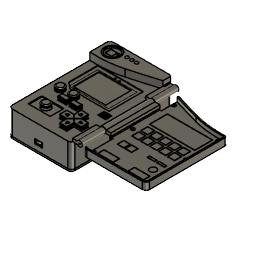
pokedexV4 (Autodesk Fusion 360 design; units mm, degrees)
part number: 2026-07-24-11-06-57-032
Autodesk Fusion 360 part; units mm, degrees
(part 1 of 3)
sketch "TubOutline" plane through (0, 0, 0) normal (0, 0, 1) x (1, 0, 0)
  line L0 (0, 0) -> (105, 0)
  line L1 (105, 0) -> (105, 170)
  line L2 (105, 170) -> (0, 170)
  line L3 (0, 170) -> (0, 0)
extrude "Extrude38" add sketch "TubOutline" against normal blind 44 makes body 1
fillet "Fillet13" radius 6 4 edges at (0, 0, -22) (105, 0, -22) (105, 170, -22) (0, 170, -22) on bodies 1
sketch "ShoulderStep" plane through (0, 0, 0) normal (0, 0, 1) x (1, 0, 0)
  arc A0 (0, 136) -> (54, 141) centre (11.7114, 303.6168) ccw
  arc A1 (54, 141) -> (105, 156) centre (-358, 1636) ccw
  line L0 (105, 156) -> (105, 0)
  line L1 (105, 0) -> (0, 0)
  line L2 (0, 0) -> (0, 136)
extrude "Extrude39" cut sketch "ShoulderStep" against normal blind 4 bodies 1
shell "Shell6" thickness 2.4 removed faces 1 at (35, 111.3333, -44) on bodies 1
ref_plane "WorkPlane4" through (0, 0, -4) normal (0, 0, 1) x (1, 0, 0)
sketch "FaceCuts" plane through (0, 0, -4) normal (0, 0, 1) x (1, 0, 0)
  line L0 (21.2, 84.4) -> (78.8, 84.4)
  line L1 (78.8, 84.4) -> (78.8, 127.6)
  line L2 (78.8, 127.6) -> (21.2, 127.6)
  line L3 (21.2, 127.6) -> (21.2, 84.4)
  line L4 (12.7, 75.9) -> (87.3, 75.9)
  line L5 (87.3, 75.9) -> (87.3, 136.1)
  line L6 (87.3, 136.1) -> (12.7, 136.1)
  line L7 (12.7, 136.1) -> (12.7, 75.9)
  circle A0 centre (17.5, 69) radius 7.2
  line L8 (65.5, 63) -> (88.5, 63)
  line L9 (88.5, 63) -> (88.5, 64.5)
  line L10 (88.5, 64.5) -> (65.5, 64.5)
  line L11 (65.5, 64.5) -> (65.5, 63)
  line L12 (65.5, 66) -> (88.5, 66)
  line L13 (88.5, 66) -> (88.5, 67.5)
  line L14 (88.5, 67.5) -> (65.5, 67.5)
  line L15 (65.5, 67.5) -> (65.5, 66)
  line L16 (65.5, 69) -> (88.5, 69)
  line L17 (88.5, 69) -> (88.5, 70.5)
  line L18 (88.5, 70.5) -> (65.5, 70.5)
  line L19 (65.5, 70.5) -> (65.5, 69)
  line L20 (65.5, 72) -> (88.5, 72)
  line L21 (88.5, 72) -> (88.5, 73.5)
  line L22 (88.5, 73.5) -> (65.5, 73.5)
  line L23 (65.5, 73.5) -> (65.5, 72)
  line L24 (65.5, 75) -> (88.5, 75)
  line L25 (88.5, 75) -> (88.5, 76.5)
  line L26 (88.5, 76.5) -> (65.5, 76.5)
  line L27 (65.5, 76.5) -> (65.5, 75)
  line L28 (65.5, 78) -> (88.5, 78)
  line L29 (88.5, 78) -> (88.5, 79.5)
  line L30 (88.5, 79.5) -> (65.5, 79.5)
  line L31 (65.5, 79.5) -> (65.5, 78)
  line L32 (65.5, 81) -> (88.5, 81)
  line L33 (88.5, 81) -> (88.5, 82.5)
  line L34 (88.5, 82.5) -> (65.5, 82.5)
  line L35 (65.5, 82.5) -> (65.5, 81)
  line L36 (30.5, 54) -> (45.5, 54)
  line L37 (45.5, 54) -> (45.5, 58)
  line L38 (45.5, 58) -> (30.5, 58)
  line L39 (30.5, 58) -> (30.5, 54)
  line L40 (49.5, 54) -> (64.5, 54)
  line L41 (64.5, 54) -> (64.5, 58)
  line L42 (64.5, 58) -> (49.5, 58)
  line L43 (49.5, 58) -> (49.5, 54)
  line L44 (11.5, 21) -> (48.5, 21)
  line L45 (48.5, 21) -> (48.5, 44)
  line L46 (48.5, 44) -> (11.5, 44)
  line L47 (11.5, 44) -> (11.5, 21)
  line L48 (71.3, 13.5) -> (83.7, 13.5)
  line L49 (83.7, 13.5) -> (83.7, 50.5)
  line L50 (83.7, 50.5) -> (71.3, 50.5)
  line L51 (71.3, 50.5) -> (71.3, 13.5)
  line L52 (59, 25.8) -> (96, 25.8)
  line L53 (96, 25.8) -> (96, 38.2)
  line L54 (96, 38.2) -> (59, 38.2)
  line L55 (59, 38.2) -> (59, 25.8)
extrude "Extrude40" cut sketch "FaceCuts" against normal blind 1.6 contours L0 L1 L2 L3 | L4 L5 L6 L7 A0 L26 L27 L28 L30 L31 L32 L34 L35 bodies 1
extrude "Extrude41" cut sketch "FaceCuts" against normal blind 6 contours L0 L1 L2 L3 bodies 1
extrude "Extrude42" cut sketch "FaceCuts" against normal blind 6 contours L4 A0 picked at (17.378, 71.2031) bodies 1
extrude "Extrude43" cut sketch "FaceCuts" against normal blind 6 contours L4 L5 L26 L27 | L4 L5 L24 L25 L26 L27 | L5 L32 L33 L34 | L5 L32 L34 L35 | L5 L28 L29 L30 | L5 L28 L30 L31 | L8 L9 L10 L11 | L12 L13 L14 L15 | L16 L17 L18 L19 | L20 L21 L22 L23 bodies 1
extrude "Extrude44" cut sketch "FaceCuts" against normal blind 6 contours L36 L37 L38 L39 | L40 L41 L42 L43 bodies 1
extrude "Extrude45" cut sketch "FaceCuts" against normal blind 1.6 contours L44 L45 L46 L47 bodies 1
extrude "Extrude46" cut sketch "FaceCuts" against normal blind 6 contours L48 L49 L51 L52 | L51 L52 L54 L55 | L49 L51 L52 L54 | L49 L52 L53 L54 | L49 L50 L51 L54 bodies 1
sketch "ShoulderDetail" plane through (0, 0, 0) normal (0, 0, 1) x (1, 0, 0)
  circle A0 centre (19, 155) radius 13.5
  circle A1 centre (39, 159.5) radius 2.8
  circle A2 centre (47, 159.5) radius 2.8
  circle A3 centre (55, 159.5) radius 2.8
extrude "Extrude47" cut sketch "ShoulderDetail" against normal blind 2.2 contours A0 bodies 1
extrude "Extrude48" cut sketch "ShoulderDetail" against normal blind 8 contours A1 | A2 | A3 bodies 1
ref_plane "WorkPlane5" through (0, 0, -6.4) normal (0, 0, 1) x (1, 0, 0)
sketch "PlateBosses" plane through (0, 0, -6.4) normal (0, 0, 1) x (1, 0, 0)
  circle A0 centre (11.5, 11.5) radius 4.2
  circle A1 centre (11.5, 85) radius 4.2
  circle A2 centre (11.5, 156) radius 4.2
  circle A3 centre (93, 11.5) radius 4.2
  circle A4 centre (93, 80) radius 4.2
  circle A5 centre (93, 120) radius 4.2
extrude "Extrude51" add sketch "PlateBosses" against normal blind 37.6 bodies 1 makes body 2 at (14.7174, 158.6997, -31.4667)
sketch "PlatePilots" plane through (0, 0, -6.4) normal (0, 0, 1) x (1, 0, 0)
  circle A0 centre (11.5, 11.5) radius 1.25
  circle A1 centre (11.5, 85) radius 1.25
  circle A2 centre (11.5, 156) radius 1.25
  circle A3 centre (93, 11.5) radius 1.25
  circle A4 centre (93, 80) radius 1.25
  circle A5 centre (93, 120) radius 1.25
extrude "Extrude52" cut sketch "PlatePilots" against normal blind 12 from surface at -26 bodies 1
sketch "USBC" plane through (0, 0, 0) normal (0, 1, 0) x (1, 0, 0)
  line L0 (45.5, 28) -> (54.5, 28)
  line L1 (54.5, 28) -> (54.5, 31.5)
  line L2 (54.5, 31.5) -> (45.5, 31.5)
  line L3 (45.5, 31.5) -> (45.5, 28)
extrude "Extrude53" cut sketch "USBC" along normal mid plane 16 bodies 1
ref_plane "WorkPlane6" through (0, 0, -44) normal (0, 0, 1) x (1, 0, 0)
sketch "PlateOutline" plane through (0, 0, -44) normal (0, 0, 1) x (1, 0, 0)
  line L0 (0, 0) -> (105, 0)
  line L1 (105, 0) -> (105, 170)
  line L2 (105, 170) -> (0, 170)
  line L3 (0, 170) -> (0, 0)
extrude "Extrude60" add sketch "PlateOutline" against normal blind 3 separate body makes body 3
fillet "Fillet15" radius 6 4 edges at (0, 0, -45.5) (105, 0, -45.5) (105, 170, -45.5) (0, 170, -45.5) on bodies 3
sketch "PlateFeatures" plane through (0, 0, -44) normal (0, 0, 1) x (1, 0, 0)
  circle A0 centre (11.5, 11.5) radius 1.6
  circle A1 centre (11.5, 85) radius 1.6
  circle A2 centre (11.5, 156) radius 1.6
  circle A3 centre (93, 11.5) radius 1.6
  circle A4 centre (93, 80) radius 1.6
  circle A5 centre (93, 120) radius 1.6
  circle A6 centre (52, 132) radius 21
  line L0 (47.5, 127.5) -> (56.5, 127.5)
  line L1 (56.5, 127.5) -> (56.5, 136.5)
  line L2 (56.5, 136.5) -> (47.5, 136.5)
  line L3 (47.5, 136.5) -> (47.5, 127.5)
extrude "Extrude61" cut sketch "PlateFeatures" against normal blind 4 contours A0 | A1 | A2 | A3 | A4 | A5 bodies 3
extrude "Extrude62" cut sketch "PlateFeatures" against normal blind 1 contours A6 bodies 3
extrude "Extrude63" cut sketch "PlateFeatures" against normal blind 4 contours L0 L1 L2 L3 bodies 3
sketch "BossBridge" plane through (0, 0, 0) normal (0, 0, 1) x (1, 0, 0)
  circle A0 centre (11.5, 156) radius 4.2
extrude "Extrude66" add sketch "BossBridge" against normal blind 5 from surface at -2 bodies 1 2
sketch "FillVoids" plane through (0, 0, 0) normal (0, 0, 1) x (1, 0, 0)
  circle A0 centre (19, 155) radius 13.5
  circle A1 centre (39, 159.5) radius 2.8
  circle A2 centre (47, 159.5) radius 2.8
  circle A3 centre (55, 159.5) radius 2.8
extrude "Extrude75" add sketch "FillVoids" along normal blind 8 from surface at -8 bodies 1
sketch "ShoulderRaise" plane through (0, 0, 0) normal (0, 0, 1) x (1, 0, 0)
  arc A0 (0, 136) -> (54, 141) centre (11.7114, 303.6168) ccw
  arc A1 (54, 141) -> (105, 156) centre (-358, 1636) ccw
  line L0 (105, 156) -> (105, 164)
  arc A2 (105, 164) -> (99, 170) centre (98.991, 163.991) ccw
  line L1 (99, 170) -> (6, 170)
  arc A3 (6, 170) -> (0, 164) centre (6.009, 163.991) ccw
  line L2 (0, 164) -> (0, 136)
extrude "Extrude76" add sketch "ShoulderRaise" along normal blind 8 bodies 1
ref_plane "WorkPlane7" through (0, 0, 8) normal (0, 0, 1) x (1, 0, 0)
sketch "ShoulderDetail2" plane through (0, 0, 8) normal (0, 0, 1) x (1, 0, 0)
  circle A0 centre (19, 155) radius 13.5
  circle A1 centre (39, 159.5) radius 2.8
  circle A2 centre (47, 159.5) radius 2.8
  circle A3 centre (55, 159.5) radius 2.8
extrude "Extrude77" cut sketch "ShoulderDetail2" against normal blind 2.2 contours A0 bodies 1
extrude "Extrude78" cut sketch "ShoulderDetail2" against normal blind 16 contours A1 | A2 | A3 bodies 1
sketch "SwingRelief" plane through (0, 0, 0) normal (0, 1, 0) x (1, 0, 0)
  line L0 (103.2, -8.5) -> (105.5, -8.5)
  line L1 (105.5, -8.5) -> (105.5, -0.5)
  line L2 (105.5, -0.5) -> (103.2, -0.5)
  line L3 (103.2, -0.5) -> (103.2, -8.5)
extrude "Extrude88" cut sketch "SwingRelief" along normal blind 42 from surface at 128 bodies 1
sketch "LidOutline" plane through (0, 0, 0) normal (0, 0, 1) x (1, 0, 0)
  arc A0 (125, 156) -> (176, 141) centre (588, 1636) ccw
  arc A1 (176, 141) -> (230, 136) centre (218.2886, 303.6168) ccw
  line L0 (230, 136) -> (230, 0)
  line L1 (230, 0) -> (125, 0)
  line L2 (125, 0) -> (125, 156)
extrude "Extrude89" add sketch "LidOutline" against normal blind 12 separate body makes body 4
fillet "Fillet19" radius 6 2 edges at (230, 0, -6) (125, 0, -6) on bodies 4
fillet "Fillet20" radius 3 1 edges at (230, 136, -6) on bodies 4
shell "Shell10" thickness 2.4 removed faces 1 at (182.5811, 49.8482, 0) on bodies 4
ref_plane "WorkPlane8" through (0, 0, -2) normal (0, 0, 1) x (1, 0, 0)
sketch "LidBosses" plane through (0, 0, -2) normal (0, 0, 1) x (1, 0, 0)
  circle A0 centre (133, 9) radius 3.2
  circle A1 centre (133, 75) radius 3.2
  circle A2 centre (133, 144) radius 3.2
  circle A3 centre (222, 9) radius 3.2
  circle A4 centre (222, 75) radius 3.2
  circle A5 centre (222, 129) radius 3.2
extrude "Extrude95" add sketch "LidBosses" against normal blind 10 bodies 4
sketch "LidInsertBores" plane through (0, 0, -2) normal (0, 0, 1) x (1, 0, 0)
  circle A0 centre (133, 9) radius 1.6
  circle A1 centre (133, 75) radius 1.6
  circle A2 centre (133, 144) radius 1.6
  circle A3 centre (222, 9) radius 1.6
  circle A4 centre (222, 75) radius 1.6
  circle A5 centre (222, 129) radius 1.6
extrude "Extrude96" cut sketch "LidInsertBores" against normal blind 4.5 bodies 4
sketch "FacePlateOutline" plane through (0, 0, 0) normal (0, 0, 1) x (1, 0, 0)
  arc A0 (127.9, 152.5) -> (176, 138.5) centre (719.1151, 2094.1174) ccw
  arc A1 (176, 138.5) -> (227.1, 133.5) centre (217.0513, 294.4236) ccw
  line L0 (227.1, 133.5) -> (227.1, 2.9)
  line L1 (227.1, 2.9) -> (127.9, 2.9)
  line L2 (127.9, 2.9) -> (127.9, 152.5)
extrude "Extrude97" add sketch "FacePlateOutline" along normal blind 2 from surface at -2 separate body makes body 5
sketch "FacePlateCuts" plane through (0, 0, 0) normal (0, 0, 1) x (1, 0, 0)
  line L0 (140, 96) -> (216, 96)
  line L1 (216, 96) -> (216, 126)
  line L2 (216, 126) -> (140, 126)
  line L3 (140, 126) -> (140, 96)
  line L4 (142, 79) -> (154, 79)
  line L5 (154, 79) -> (154, 91)
  line L6 (154, 91) -> (142, 91)
  line L7 (142, 91) -> (142, 79)
  line L8 (157, 79) -> (169, 79)
  line L9 (169, 79) -> (169, 91)
  line L10 (169, 91) -> (157, 91)
  line L11 (157, 91) -> (157, 79)
  line L12 (172, 79) -> (184, 79)
  line L13 (184, 79) -> (184, 91)
  line L14 (184, 91) -> (172, 91)
  line L15 (172, 91) -> (172, 79)
  line L16 (187, 79) -> (199, 79)
  line L17 (199, 79) -> (199, 91)
  line L18 (199, 91) -> (187, 91)
  line L19 (187, 91) -> (187, 79)
  line L20 (202, 79) -> (214, 79)
  line L21 (214, 79) -> (214, 91)
  line L22 (214, 91) -> (202, 91)
  line L23 (202, 91) -> (202, 79)
  line L24 (142, 64) -> (154, 64)
  line L25 (154, 64) -> (154, 76)
  line L26 (154, 76) -> (142, 76)
  line L27 (142, 76) -> (142, 64)
  line L28 (157, 64) -> (169, 64)
  line L29 (169, 64) -> (169, 76)
  line L30 (169, 76) -> (157, 76)
  line L31 (157, 76) -> (157, 64)
  line L32 (172, 64) -> (184, 64)
  line L33 (184, 64) -> (184, 76)
  line L34 (184, 76) -> (172, 76)
  line L35 (172, 76) -> (172, 64)
  line L36 (187, 64) -> (199, 64)
  line L37 (199, 64) -> (199, 76)
  line L38 (199, 76) -> (187, 76)
  line L39 (187, 76) -> (187, 64)
  line L40 (202, 64) -> (214, 64)
  line L41 (214, 64) -> (214, 76)
  line L42 (214, 76) -> (202, 76)
  line L43 (202, 76) -> (202, 64)
  line L44 (142, 40) -> (153, 40)
  line L45 (153, 40) -> (153, 51)
  line L46 (153, 51) -> (142, 51)
  line L47 (142, 51) -> (142, 40)
  line L48 (155, 40) -> (166, 40)
  line L49 (166, 40) -> (166, 51)
  line L50 (166, 51) -> (155, 51)
  line L51 (155, 51) -> (155, 40)
  line L52 (186, 46) -> (199, 46)
  line L53 (199, 46) -> (199, 50)
  line L54 (199, 50) -> (186, 50)
  line L55 (186, 50) -> (186, 46)
  line L56 (202, 46) -> (215, 46)
  line L57 (215, 46) -> (215, 50)
  line L58 (215, 50) -> (202, 50)
  line L59 (202, 50) -> (202, 46)
  circle A0 centre (209, 33) radius 5.5
  line L60 (139, 10) -> (165, 10)
  line L61 (165, 10) -> (165, 21)
  line L62 (165, 21) -> (139, 21)
  line L63 (139, 21) -> (139, 10)
  line L64 (190, 10) -> (216, 10)
  line L65 (216, 10) -> (216, 21)
  line L66 (216, 21) -> (190, 21)
  line L67 (190, 21) -> (190, 10)
  circle A1 centre (133, 9) radius 1.15
  circle A2 centre (133, 75) radius 1.15
  circle A3 centre (133, 144) radius 1.15
  circle A4 centre (222, 9) radius 1.15
  circle A5 centre (222, 75) radius 1.15
  circle A6 centre (222, 129) radius 1.15
extrude "Extrude98" cut sketch "FacePlateCuts" along normal blind 3 from surface at -2.5 bodies 5
ref_plane "WorkPlane9" through (0, 0, -44) normal (0, 0, 1) x (1, 0, 0)
sketch "M3Bores" plane through (0, 0, -44) normal (0, 0, 1) x (1, 0, 0)
  circle A0 centre (11.5, 11.5) radius 2
  circle A1 centre (11.5, 85) radius 2
  circle A2 centre (11.5, 156) radius 2
  circle A3 centre (93, 11.5) radius 2
  circle A4 centre (93, 80) radius 2
  circle A5 centre (93, 120) radius 2
extrude "Extrude99" cut sketch "M3Bores" along normal blind 6.5 bodies 1
sketch "M3Clear" plane through (0, 0, -44) normal (0, 0, 1) x (1, 0, 0)
  circle A0 centre (11.5, 11.5) radius 1.7
  circle A1 centre (11.5, 85) radius 1.7
  circle A2 centre (11.5, 156) radius 1.7
  circle A3 centre (93, 11.5) radius 1.7
  circle A4 centre (93, 80) radius 1.7
  circle A5 centre (93, 120) radius 1.7
extrude "Extrude100" cut sketch "M3Clear" against normal blind 4 bodies 3
sketch "LidNotches" plane through (0, 0, 0) normal (0, 0, 1) x (1, 0, 0)
  line L0 (124.5, 3) -> (130.5, 3)
  line L1 (130.5, 3) -> (130.5, 44.5)
  line L2 (130.5, 44.5) -> (124.5, 44.5)
  line L3 (124.5, 44.5) -> (124.5, 3)
  line L4 (124.5, 125.5) -> (130.5, 125.5)
  line L5 (130.5, 125.5) -> (130.5, 157)
  line L6 (130.5, 157) -> (124.5, 157)
  line L7 (124.5, 157) -> (124.5, 125.5)
extrude "Extrude108" cut sketch "LidNotches" against normal blind 16 from surface at 2 bodies 4
extrude "Extrude109" cut sketch "LidNotches" against normal blind 3 from surface at 0.5 bodies 5
sketch "SpineTrim" plane through (0, 0, 0) normal (0, 1, 0) x (1, 0, 0)
  line L0 (103.5, 0) -> (105.5, 0)
  line L1 (105.5, 0) -> (105.5, 2.5)
  line L2 (105.5, 2.5) -> (103.5, 2.5)
  line L3 (103.5, 2.5) -> (103.5, 0)
extrude "Extrude110" cut sketch "SpineTrim" along normal blind 156 from surface at 4 bodies 1
sketch "WindowEnlarge" plane through (0, 0, 0) normal (0, 0, 1) x (1, 0, 0)
  line L0 (20.7, 83.9) -> (79.3, 83.9)
  line L1 (79.3, 83.9) -> (79.3, 128.1)
  line L2 (79.3, 128.1) -> (20.7, 128.1)
  line L3 (20.7, 128.1) -> (20.7, 83.9)
extrude "Extrude111" cut sketch "WindowEnlarge" against normal blind 8 bodies 1
sketch "LCDPocketRibs" plane through (0, 0, -6.4) normal (0, 0, 1) x (1, 0, 0)
  line L0 (15.95, 78.55) -> (18.95, 78.55)
  line L1 (18.95, 78.55) -> (18.95, 130.45)
  line L2 (18.95, 130.45) -> (15.95, 130.45)
  line L3 (15.95, 130.45) -> (15.95, 78.55)
  line L4 (85.65, 78.55) -> (88.65, 78.55)
  line L5 (88.65, 78.55) -> (88.65, 130.45)
  line L6 (88.65, 130.45) -> (85.65, 130.45)
  line L7 (85.65, 130.45) -> (85.65, 78.55)
  line L8 (15.95, 78.55) -> (88.65, 78.55)
  line L9 (88.65, 78.55) -> (88.65, 81.55)
  line L10 (88.65, 81.55) -> (15.95, 81.55)
  line L11 (15.95, 81.55) -> (15.95, 78.55)
  line L12 (15.95, 139.05) -> (27.95, 139.05)
  line L13 (27.95, 139.05) -> (27.95, 142.05)
  line L14 (27.95, 142.05) -> (15.95, 142.05)
  line L15 (15.95, 142.05) -> (15.95, 139.05)
  line L16 (76.65, 139.05) -> (88.65, 139.05)
  line L17 (88.65, 139.05) -> (88.65, 142.05)
  line L18 (88.65, 142.05) -> (76.65, 142.05)
  line L19 (76.65, 142.05) -> (76.65, 139.05)
extrude "Extrude112" add sketch "LCDPocketRibs" against normal blind 10 bodies 1
sketch "ClampPedestals" plane through (0, 0, -6.4) normal (0, 0, 1) x (1, 0, 0)
  circle A0 centre (11.5, 106) radius 4
  circle A1 centre (93.5, 106) radius 4
extrude "Extrude113" add sketch "ClampPedestals" against normal blind 8 bodies 1
sketch "ClampInsertBores" plane through (0, 0, -6.4) normal (0, 0, 1) x (1, 0, 0)
  circle A0 centre (11.5, 106) radius 1.6
  circle A1 centre (93.5, 106) radius 1.6
extrude "Extrude114" cut sketch "ClampInsertBores" against normal blind 4.5 from surface at -3.5 bodies 1
ref_plane "WorkPlane10" through (0, 0, -14.4) normal (0, 0, 1) x (1, 0, 0)
ref_plane "WorkPlane11" through (0, 0, -13.6) normal (0, 0, 1) x (1, 0, 0)
sketch "CrossPlateOutline" plane through (0, 0, -13.6) normal (0, 0, 1) x (1, 0, 0)
  line L0 (16, 105.5) -> (88.6, 105.5)
  line L1 (88.6, 105.5) -> (88.6, 139.5)
  line L2 (88.6, 139.5) -> (16, 139.5)
  line L3 (16, 139.5) -> (16, 105.5)
extrude "Extrude117" add sketch "CrossPlateOutline" against normal blind 2.5 separate body makes body 6
sketch "CrossPlateCuts" plane through (0, 0, -13.6) normal (0, 0, 1) x (1, 0, 0)
  circle A0 centre (24.05, 134.1) radius 2.8
  circle A1 centre (82.05, 134.1) radius 2.8
  circle A2 centre (24.05, 111.1) radius 2.8
  circle A3 centre (82.05, 111.1) radius 2.8
  line L0 (33, 107.5) -> (73, 107.5)
  line L1 (73, 107.5) -> (73, 137.5)
  line L2 (73, 137.5) -> (33, 137.5)
  line L3 (33, 137.5) -> (33, 107.5)
extrude "Extrude118" cut sketch "CrossPlateCuts" against normal blind 3 bodies 6
sketch "PedestalExtend" plane through (0, 0, -6.4) normal (0, 0, 1) x (1, 0, 0)
  circle A0 centre (11.5, 106) radius 4
  circle A1 centre (93.5, 106) radius 4
extrude "Extrude119" add sketch "PedestalExtend" against normal blind 10 bodies 1
sketch "PedestalBores2" plane through (0, 0, -6.4) normal (0, 0, 1) x (1, 0, 0)
  circle A0 centre (11.5, 106) radius 1.6
  circle A1 centre (93.5, 106) radius 1.6
extrude "Extrude120" cut sketch "PedestalBores2" against normal blind 4.5 from surface at -5.5 bodies 1
sketch "PlateEars" plane through (0, 0, -13.6) normal (0, 0, 1) x (1, 0, 0)
  line L0 (7, 101) -> (16.2, 101)
  line L1 (16.2, 101) -> (16.2, 111)
  line L2 (16.2, 111) -> (7, 111)
  line L3 (7, 111) -> (7, 101)
  line L4 (88.4, 101) -> (98, 101)
  line L5 (98, 101) -> (98, 111)
  line L6 (98, 111) -> (88.4, 111)
  line L7 (88.4, 111) -> (88.4, 101)
extrude "Extrude121" add sketch "PlateEars" against normal blind 2.5 bodies 6
sketch "EarHoles" plane through (0, 0, -13.6) normal (0, 0, 1) x (1, 0, 0)
  circle A0 centre (11.5, 106) radius 1.15
  circle A1 centre (93.5, 106) radius 1.15
extrude "Extrude122" cut sketch "EarHoles" against normal blind 3 bodies 6
sketch "HoleFill" plane through (0, 0, -13.6) normal (0, 0, 1) x (1, 0, 0)
  circle A0 centre (24.05, 134.1) radius 2.85
  circle A1 centre (82.05, 134.1) radius 2.85
  circle A2 centre (24.05, 111.1) radius 2.85
  circle A3 centre (82.05, 111.1) radius 2.85
extrude "Extrude123" add sketch "HoleFill" against normal blind 2.5 bodies 6
sketch "M25Holes" plane through (0, 0, -13.6) normal (0, 0, 1) x (1, 0, 0)
  circle A0 centre (24.05, 134.1) radius 1.35
  circle A1 centre (82.05, 134.1) radius 1.35
  circle A2 centre (24.05, 111.1) radius 1.35
  circle A3 centre (82.05, 111.1) radius 1.35
extrude "Extrude124" cut sketch "M25Holes" against normal blind 3 bodies 6
sketch "HingeTub" plane through (0, 0, 0) normal (0, 1, 0) x (1, 0, 0)
  circle A0 centre (115, 2) radius 4.5
  line L0 (103, 0) -> (115, 0)
  line L1 (115, 0) -> (115, 5)
  line L2 (115, 5) -> (103, 5)
  line L3 (103, 5) -> (103, 0)
extrude "Extrude125" add sketch "HingeTub" along normal blind 39.7 from surface at 4 bodies 1
extrude "Extrude126" add sketch "HingeTub" along normal blind 39.7 from surface at 126.3 bodies 1
sketch "HingeLid" plane through (0, 0, 0) normal (0, 1, 0) x (1, 0, 0)
  circle A0 centre (115, 2) radius 4.5
  line L0 (115, 0) -> (128, 0)
  line L1 (128, 0) -> (128, 5)
  line L2 (128, 5) -> (115, 5)
  line L3 (115, 5) -> (115, 0)
extrude "Extrude127" add sketch "HingeLid" along normal blind 82 from surface at 44 bodies 4
sketch "PinBore" plane through (0, 0, 0) normal (0, 1, 0) x (1, 0, 0)
  circle A0 centre (115, 2) radius 1
extrude "Extrude128" cut sketch "PinBore" along normal blind 162 from surface at 4 bodies 1 4
sketch "FlushCleanup" plane through (0, 0, -13.6) normal (0, 0, 1) x (1, 0, 0)
  line L0 (15, 78) -> (89, 78)
  line L1 (89, 78) -> (89, 140)
  line L2 (89, 140) -> (15, 140)
  line L3 (15, 140) -> (15, 78)
extrude "Extrude129" cut sketch "FlushCleanup" against normal blind 8 bodies 1
sketch "PedestalBoresFlush" plane through (0, 0, -13.6) normal (0, 0, 1) x (1, 0, 0)
  circle A0 centre (11.5, 106) radius 1.6
  circle A1 centre (93.5, 106) radius 1.6
extrude "Extrude130" cut sketch "PedestalBoresFlush" along normal blind 4.5 bodies 1
ref_plane "WorkPlane12" through (0, 0, -5.6) normal (0, 0, 1) x (1, 0, 0)
sketch "DisplayDummySk" plane through (0, 0, -5.6) normal (0, 0, 1) x (1, 0, 0)
  line L0 (19.45, 82.05) -> (85.15, 82.05)
  line L1 (85.15, 82.05) -> (85.15, 129.95)
  line L2 (85.15, 129.95) -> (19.45, 129.95)
  line L3 (19.45, 129.95) -> (19.45, 82.05)
extrude "Extrude132" add sketch "DisplayDummySk" against normal blind 8 separate body makes body 7
sketch "KnuckleGap" plane through (0, 0, 0) normal (0, 1, 0) x (1, 0, 0)
  line L0 (109, -8) -> (124.9, -8)
  line L1 (124.9, -8) -> (124.9, 8)
  line L2 (124.9, 8) -> (109, 8)
  line L3 (109, 8) -> (109, -8)
extrude "Extrude133" cut sketch "KnuckleGap" along normal blind 16 from surface at 77 bodies 4
sketch "WireSlot" plane through (0, 0, 0) normal (1, 0, 0) x (0, 0, -1)
  line L0 (3, 79.5) -> (11, 79.5)
  line L1 (11, 79.5) -> (11, 90.5)
  line L2 (11, 90.5) -> (3, 90.5)
  line L3 (3, 90.5) -> (3, 79.5)
extrude "Extrude134" cut sketch "WireSlot" along normal blind 6 from surface at 102 bodies 1
extrude "Extrude135" cut sketch "WireSlot" along normal blind 6 from surface at 124 bodies 4
sketch "PokeballFill" plane through (0, 0, -44) normal (0, 0, 1) x (1, 0, 0)
  circle A0 centre (52, 132) radius 21
  line L0 (47.5, 127.5) -> (56.5, 127.5)
  line L1 (56.5, 127.5) -> (56.5, 136.5)
  line L2 (56.5, 136.5) -> (47.5, 136.5)
  line L3 (47.5, 136.5) -> (47.5, 127.5)
extrude "Extrude138" add sketch "PokeballFill" against normal blind 1 bodies 3
ref_plane "WorkPlane13" through (0, 0, -47) normal (0, 0, 1) x (1, 0, 0)
sketch "PokeballOuter" plane through (0, 0, -47) normal (0, 0, 1) x (1, 0, 0)
  circle A0 centre (52, 132) radius 21
  line L0 (47.5, 127.5) -> (56.5, 127.5)
  line L1 (56.5, 127.5) -> (56.5, 136.5)
  line L2 (56.5, 136.5) -> (47.5, 136.5)
  line L3 (47.5, 136.5) -> (47.5, 127.5)
extrude "Extrude139" cut sketch "PokeballOuter" along normal blind 1 bodies 3
sketch "RingRibs" plane through (0, 0, -47) normal (0, 0, 1) x (1, 0, 0)
  circle A0 centre (52, 132) radius 21
  line L0 (47.5, 127.5) -> (56.5, 127.5)
  line L1 (56.5, 127.5) -> (56.5, 136.5)
  line L2 (56.5, 136.5) -> (47.5, 136.5)
  line L3 (47.5, 136.5) -> (47.5, 127.5)
  line L4 (29, 137.6) -> (75, 137.6)
  line L5 (75, 137.6) -> (75, 139.2)
  line L6 (75, 139.2) -> (29, 139.2)
  line L7 (29, 139.2) -> (29, 137.6)
  line L8 (29, 140.8) -> (75, 140.8)
  line L9 (75, 140.8) -> (75, 142.4)
  line L10 (75, 142.4) -> (29, 142.4)
  line L11 (29, 142.4) -> (29, 140.8)
  line L12 (29, 144) -> (75, 144)
  line L13 (75, 144) -> (75, 145.6)
  line L14 (75, 145.6) -> (29, 145.6)
  line L15 (29, 145.6) -> (29, 144)
  line L16 (29, 147.2) -> (75, 147.2)
  line L17 (75, 147.2) -> (75, 148.8)
  line L18 (75, 148.8) -> (29, 148.8)
  line L19 (29, 148.8) -> (29, 147.2)
  line L20 (29, 150.4) -> (75, 150.4)
  line L21 (75, 150.4) -> (75, 152)
  line L22 (75, 152) -> (29, 152)
  line L23 (29, 152) -> (29, 150.4)
  line L24 (29, 124.8) -> (75, 124.8)
  line L25 (75, 124.8) -> (75, 126.4)
  line L26 (75, 126.4) -> (29, 126.4)
  line L27 (29, 126.4) -> (29, 124.8)
  line L28 (29, 121.6) -> (75, 121.6)
  line L29 (75, 121.6) -> (75, 123.2)
  line L30 (75, 123.2) -> (29, 123.2)
  line L31 (29, 123.2) -> (29, 121.6)
  line L32 (29, 118.4) -> (75, 118.4)
  line L33 (75, 118.4) -> (75, 120)
  line L34 (75, 120) -> (29, 120)
  line L35 (29, 120) -> (29, 118.4)
  line L36 (29, 115.2) -> (75, 115.2)
  line L37 (75, 115.2) -> (75, 116.8)
  line L38 (75, 116.8) -> (29, 116.8)
  line L39 (29, 116.8) -> (29, 115.2)
  line L40 (29, 112) -> (75, 112)
  line L41 (75, 112) -> (75, 113.6)
  line L42 (75, 113.6) -> (29, 113.6)
  line L43 (29, 113.6) -> (29, 112)
extrude "Extrude142" add sketch "RingRibs" along normal blind 1 contours A0 L4 L6 | A0 L24 L26 | A0 L8 L10 | A0 L28 L30 | A0 L12 L14 | A0 L32 L34 | A0 L16 L18 | A0 L36 L38 | A0 L20 L22 | A0 L40 L42 bodies 3
sketch "CamShoulder" plane through (0, 0, -44) normal (0, 0, 1) x (1, 0, 0)
  circle A0 centre (32.7, 134.65) radius 3
  circle A1 centre (82.7, 134) radius 3
  circle A2 centre (82.7, 130) radius 3
extrude "Extrude147" add sketch "CamShoulder" along normal blind 2.45 bodies 3
sketch "CenterPad" plane through (0, 0, -47) normal (0, 0, 1) x (1, 0, 0)
  circle A0 centre (52, 132) radius 21
  line L0 (47.5, 127.5) -> (56.5, 127.5)
  line L1 (56.5, 127.5) -> (56.5, 136.5)
  line L2 (56.5, 136.5) -> (47.5, 136.5)
  line L3 (47.5, 136.5) -> (47.5, 127.5)
  line L4 (29, 128.5) -> (75, 128.5)
  line L5 (75, 128.5) -> (75, 135.5)
  line L6 (75, 135.5) -> (29, 135.5)
  line L7 (29, 135.5) -> (29, 128.5)
extrude "Extrude151" add sketch "CenterPad" along normal blind 1 contours A0 L1 L4 L6 | A0 L3 L4 L6 bodies 3
sketch "SinglePad" plane through (0, 0, -47) normal (0, 0, 1) x (1, 0, 0)
  circle A0 centre (52, 132) radius 21
  line L0 (29, 133) -> (37.5, 133)
  line L1 (37.5, 133) -> (37.5, 139)
  line L2 (37.5, 139) -> (29, 139)
  line L3 (29, 139) -> (29, 133)
extrude "Extrude152" add sketch "SinglePad" along normal blind 1 contours A0 L0 L1 L2 picked at (35.538, 136.3471) bodies 3
sketch "CamScrewPilots" plane through (0, 0, -44) normal (0, 0, 1) x (1, 0, 0)
  circle A0 centre (32.7, 134.65) radius 0.8
  circle A1 centre (82.7, 134) radius 0.8
  circle A2 centre (82.7, 130) radius 0.8
extrude "Extrude153" cut sketch "CamScrewPilots" against normal blind 4 from surface at 2.45 bodies 3
extrude "Extrude154" add 1 faces at (40.8333, 136.5333, -46) along direction (0, 0, -1) blind 1 on bodies 3 bodies 3
extrude "Extrude155" add 1 faces at (50.5, 126.7667, -46) along direction (0, 0, -1) blind 1 on bodies 3 bodies 3
sketch "GlassOpening" plane through (0, 0, 0) normal (0, 0, 1) x (1, 0, 0)
  line L0 (26.2, 84.8) -> (83, 84.8)
  line L1 (83, 84.8) -> (83, 127.2)
  line L2 (83, 127.2) -> (26.2, 127.2)
  line L3 (26.2, 127.2) -> (26.2, 84.8)
extrude "Extrude158" cut sketch "GlassOpening" against normal blind 8 bodies 1
sketch "BezelFill" plane through (0, 0, -4) normal (0, 0, 1) x (1, 0, 0)
  line L0 (12, 75) -> (88, 75)
  line L1 (88, 75) -> (88, 137)
  line L2 (88, 137) -> (12, 137)
  line L3 (12, 137) -> (12, 75)
  line L4 (26.2, 84.8) -> (83, 84.8)
  line L5 (83, 84.8) -> (83, 127.2)
  line L6 (83, 127.2) -> (26.2, 127.2)
  line L7 (26.2, 127.2) -> (26.2, 84.8)
extrude "Extrude159" add sketch "BezelFill" against normal blind 1.6 contours L4 L5 L6 L7 bodies 1
sketch "BezelRecess2" plane through (0, 0, -4) normal (0, 0, 1) x (1, 0, 0)
  line L0 (18.2, 76.8) -> (91, 76.8)
  line L1 (91, 76.8) -> (91, 135.2)
  line L2 (91, 135.2) -> (18.2, 135.2)
  line L3 (18.2, 135.2) -> (18.2, 76.8)
  line L4 (26.2, 84.8) -> (83, 84.8)
  line L5 (83, 84.8) -> (83, 127.2)
  line L6 (83, 127.2) -> (26.2, 127.2)
  line L7 (26.2, 127.2) -> (26.2, 84.8)
extrude "Extrude160" cut sketch "BezelRecess2" against normal blind 1.6 contours L4 L5 L6 L7 bodies 1
sketch "RecessFill2" plane through (0, 0, -4) normal (0, 0, 1) x (1, 0, 0)
  line L0 (12.7, 75.9) -> (87.3, 75.9)
  line L1 (87.3, 75.9) -> (87.3, 136.1)
  line L2 (87.3, 136.1) -> (12.7, 136.1)
  line L3 (12.7, 136.1) -> (12.7, 75.9)
  line L4 (26.2, 84.8) -> (82.4, 84.8)
  line L5 (82.4, 84.8) -> (82.4, 127.2)
  line L6 (82.4, 127.2) -> (26.2, 127.2)
  line L7 (26.2, 127.2) -> (26.2, 84.8)
extrude "Extrude162" add sketch "RecessFill2" against normal blind 1.6 bodies 1
sketch "BezelRecess3" plane through (0, 0, -4) normal (0, 0, 1) x (1, 0, 0)
  line L0 (18.2, 76.8) -> (90.4, 76.8)
  line L1 (90.4, 76.8) -> (90.4, 135.2)
  line L2 (90.4, 135.2) -> (18.2, 135.2)
  line L3 (18.2, 135.2) -> (18.2, 76.8)
  line L4 (26.2, 84.8) -> (82.4, 84.8)
  line L5 (82.4, 84.8) -> (82.4, 127.2)
  line L6 (82.4, 127.2) -> (26.2, 127.2)
  line L7 (26.2, 127.2) -> (26.2, 84.8)
extrude "Extrude163" cut sketch "BezelRecess3" against normal blind 1.6 bodies 1
sketch "SkinClean" plane through (0, 0, 0) normal (0, 0, 1) x (1, 0, 0)
  line L0 (21.2, 84.4) -> (83, 84.4)
  line L1 (83, 84.4) -> (83, 127.6)
  line L2 (83, 127.6) -> (21.2, 127.6)
  line L3 (21.2, 127.6) -> (21.2, 84.4)
extrude "Extrude165" cut sketch "SkinClean" against normal blind 1.1 from surface at -5.55 bodies 1
extrude "Extrude166" add 1 faces at (59.7667, 128.1, -5.8667) along direction (0, -1, 0) blind 0.5 on bodies 1 bodies 1
extrude "Extrude167" add 1 faces at (40.2333, 83.9, -5.8667) along direction (0, 1, 0) blind 0.5 on bodies 1 bodies 1
ref_plane "WorkPlane14" through (0, 0, -34) normal (0, 0, 1) x (1, 0, 0)
ref_plane "WorkPlane15" through (0, 0, -32.4) normal (0, 0, 1) x (1, 0, 0)
ref_plane "WorkPlane16" through (0, 0, -34) normal (0, 0, 1) x (1, 0, 0)
sketch "UnoQDummySk" plane through (0, 0, -34) normal (0, 0, 1) x (1, 0, 0)
  line L0 (4, 55) -> (72.58, 55)
  line L1 (72.58, 55) -> (72.58, 108.34)
  line L2 (72.58, 108.34) -> (4, 108.34)
  line L3 (4, 108.34) -> (4, 55)
ref_plane "WorkPlane17" through (0, 0, -32.4) normal (0, 0, 1) x (1, 0, 0)
sketch "UnoQCompSk" plane through (0, 0, -32.4) normal (0, 0, 1) x (1, 0, 0)
  line L0 (7, 58) -> (69.58, 58)
  line L1 (69.58, 58) -> (69.58, 105.34)
  line L2 (69.58, 105.34) -> (7, 105.34)
  line L3 (7, 105.34) -> (7, 58)
ref_plane "WorkPlane18" through (0, 0, -32.4) normal (0, 0, 1) x (1, 0, 0)
ref_plane "WorkPlane19" through (0, 0, -33) normal (0, 0, 1) x (1, 0, 0)
extrude "Extrude183" add 1 faces at (20.7, 98.8, -6.1333) along direction (1, 0, 0) blind 4 on bodies 1 bodies 1
sketch "UnoQBosses" plane through (0, 0, -44) normal (0, 0, 1) x (1, 0, 0)
  circle A0 centre (58.58, 105.84) radius 4
  circle A1 centre (57.28, 57.54) radius 4
  circle A2 centre (6.58, 72.74) radius 4
  circle A3 centre (6.58, 100.74) radius 4
extrude "Extrude184" add sketch "UnoQBosses" along normal blind 10 bodies 3
sketch "UnoQInsertBores" plane through (0, 0, -44) normal (0, 0, 1) x (1, 0, 0)
  circle A0 centre (58.58, 105.84) radius 2
  circle A1 centre (57.28, 57.54) radius 2
  circle A2 centre (6.58, 72.74) radius 2
  circle A3 centre (6.58, 100.74) radius 2
extrude "Extrude185" cut sketch "UnoQInsertBores" against normal blind 6.5 from surface at 10 bodies 3
ref_plane "WorkPlane20" through (0, 0, -34) normal (0, 0, 1) x (1, 0, 0)
sketch "UsbCMarker" plane through (0, 0, -34) normal (0, 0, 1) x (1, 0, 0)
  line L0 (72.6, 59) -> (76, 59)
  line L1 (76, 59) -> (76, 68)
  line L2 (76, 68) -> (72.6, 68)
  line L3 (72.6, 68) -> (72.6, 59)
sketch "NewButtonHoles" plane through (0, 0, -4) normal (0, 0, 1) x (1, 0, 0)
  circle A0 centre (40, 69) radius 7.2
  circle A1 centre (30, 32.5) radius 7.2
extrude "Extrude187" cut sketch "NewButtonHoles" against normal blind 6 bodies 1
sketch "BtnStandoffBores (1)" plane through (0, 0, -6.4) normal (0, 0, 1) x (1, 0, 0)
  circle A0 centre (11.5, 26.5) radius 1.6
  circle A1 centre (62.5, 26.5) radius 1.6
  circle A2 centre (11.5, 73.5) radius 1.6
  circle A3 centre (62.5, 73.5) radius 1.6
  circle A4 centre (61.5, 17.5) radius 1.6
  circle A5 centre (93.5, 17.5) radius 1.6
  circle A6 centre (61.5, 48.5) radius 1.6
  circle A7 centre (93.5, 48.5) radius 1.6
ref_plane "WorkPlane21" through (0, 0, -16) normal (0, 0, 1) x (1, 0, 0)
ref_plane "WorkPlane22" through (0, 0, -16) normal (0, 0, 1) x (1, 0, 0)
extrude "Extrude217" cut 1 faces at (88.5, 75.5, -4.8) along direction (-1, 0, 0) blind 4 on bodies 1 bodies 1
extrude "Extrude218" add 1 faces at (88.5, 75.5, -4.8) along direction (-1, 0, 0) blind 5 on bodies 1 bodies 1
extrude "Extrude219" add 1 faces at (88.5, 72.5, -4.8) along direction (-1, 0, 0) blind 5 on bodies 1 bodies 1
extrude "Extrude220" add 1 faces at (88.5, 69.5, -4.8) along direction (-1, 0, 0) blind 5 on bodies 1 bodies 1
extrude "Extrude221" add 1 faces at (88.5, 66.5, -4.8) along direction (-1, 0, 0) blind 5 on bodies 1 bodies 1
extrude "Extrude222" add 1 faces at (88.5, 63.5, -4.8) along direction (-1, 0, 0) blind 5 on bodies 1 bodies 1
sketch "PerfLeftDummy" plane through (0, 0, -16) normal (0, 0, 1) x (1, 0, 0)
  line L0 (3.4, 24) -> (73.4, 24)
  line L1 (73.4, 24) -> (73.4, 74)
  line L2 (73.4, 74) -> (3.4, 74)
  line L3 (3.4, 74) -> (3.4, 24)
  dimension "d1989" = 50
  dimension "d1990" = 70
  measures "d1989" distance of L0.end L1.end
  measures "d1990" distance of L1.end L2.end
extrude "Extrude235" add sketch "PerfLeftDummy" against normal blind 1.6 separate body makes body 8
sketch "PerfRightDummy" plane through (0, 0, -16) normal (0, 0, 1) x (1, 0, 0)
  line L0 (52, 14) -> (93, 14)
  line L1 (93, 14) -> (93, 58)
  line L2 (93, 58) -> (52, 58)
  line L3 (52, 58) -> (52, 14)
extrude "Extrude236" add sketch "PerfRightDummy" against normal blind 1.6 separate body makes body 9
sketch "so_9_25" plane through (0, 0, -6.4) normal (0, 0, 1) x (1, 0, 0)
  circle A0 centre (9, 25) radius 4
extrude "Extrude255" add sketch "so_9_25" against normal blind 14 bodies 1
sketch "so_48_20" plane through (0, 0, -6.4) normal (0, 0, 1) x (1, 0, 0)
  circle A0 centre (48, 20) radius 4
extrude "Extrude256" add sketch "so_48_20" against normal blind 14 bodies 1
sketch "so_7_76" plane through (0, 0, -6.4) normal (0, 0, 1) x (1, 0, 0)
  circle A0 centre (7, 76) radius 4
extrude "Extrude257" add sketch "so_7_76" against normal blind 14 bodies 1
sketch "so_60_75" plane through (0, 0, -6.4) normal (0, 0, 1) x (1, 0, 0)
  circle A0 centre (60, 75) radius 4
extrude "Extrude258" add sketch "so_60_75" against normal blind 14 bodies 1
sketch "so_54_19" plane through (0, 0, -6.4) normal (0, 0, 1) x (1, 0, 0)
  circle A0 centre (54, 19) radius 4
extrude "Extrude259" add sketch "so_54_19" against normal blind 14 bodies 1
sketch "so_91_54" plane through (0, 0, -6.4) normal (0, 0, 1) x (1, 0, 0)
  circle A0 centre (91, 54) radius 4
extrude "Extrude260" add sketch "so_91_54" against normal blind 14 bodies 1
sketch "bo_9_25" plane through (0, 0, -6.4) normal (0, 0, 1) x (1, 0, 0)
  circle A0 centre (9, 25) radius 1.6
extrude "Extrude261" cut sketch "bo_9_25" along normal blind 4.5 from surface at -14 bodies 1
sketch "bo_48_20" plane through (0, 0, -6.4) normal (0, 0, 1) x (1, 0, 0)
  circle A0 centre (48, 20) radius 1.6
extrude "Extrude262" cut sketch "bo_48_20" along normal blind 4.5 from surface at -14 bodies 1
sketch "bo_7_76" plane through (0, 0, -6.4) normal (0, 0, 1) x (1, 0, 0)
  circle A0 centre (7, 76) radius 1.6
extrude "Extrude263" cut sketch "bo_7_76" along normal blind 4.5 from surface at -14 bodies 1
sketch "bo_60_75" plane through (0, 0, -6.4) normal (0, 0, 1) x (1, 0, 0)
  circle A0 centre (60, 75) radius 1.6
extrude "Extrude264" cut sketch "bo_60_75" along normal blind 4.5 from surface at -14 bodies 1
sketch "bo_54_19" plane through (0, 0, -6.4) normal (0, 0, 1) x (1, 0, 0)
  circle A0 centre (54, 19) radius 1.6
extrude "Extrude265" cut sketch "bo_54_19" along normal blind 4.5 from surface at -14 bodies 1
sketch "bo_91_54" plane through (0, 0, -6.4) normal (0, 0, 1) x (1, 0, 0)
  circle A0 centre (91, 54) radius 1.6
extrude "Extrude266" cut sketch "bo_91_54" along normal blind 4.5 from surface at -14 bodies 1
ref_plane "WorkPlane23" through (0, 0, -6.6) normal (0, 0, 1) x (1, 0, 0)
ref_plane "WorkPlane24" through (0, 0, -6.6) normal (0, 0, 1) x (1, 0, 0)
ref_plane "WorkPlane25" through (0, 0, -6.6) normal (0, 0, 1) x (1, 0, 0)
ref_plane "WorkPlane26" through (0, 0, -6.6) normal (0, 0, 1) x (1, 0, 0)
ref_plane "WorkPlane27" through (0, 0, -6.6) normal (0, 0, 1) x (1, 0, 0)
ref_plane "WorkPlane28" through (0, 0, -16) normal (0, 0, 1) x (1, 0, 0)
ref_plane "WorkPlane29" through (0, 0, -6.6) normal (0, 0, 1) x (1, 0, 0)
ref_plane "WorkPlane30" through (0, 0, -6.6) normal (0, 0, 1) x (1, 0, 0)
ref_plane "WorkPlane31" through (0, 0, -6.6) normal (0, 0, 1) x (1, 0, 0)
ref_plane "WorkPlane32" through (0, 0, -6.6) normal (0, 0, 1) x (1, 0, 0)
ref_plane "WorkPlane33" through (0, 0, -6.4) normal (0, 0, 1) x (1, 0, 0)
ref_plane "WorkPlane34" through (0, 0, -6.4) normal (0, 0, 1) x (1, 0, 0)
ref_plane "WorkPlane35" through (0, 0, -6.4) normal (0, 0, 1) x (1, 0, 0)
ref_plane "WorkPlane36" through (0, 0, -6.4) normal (0, 0, 1) x (1, 0, 0)
ref_plane "WorkPlane37" through (0, 0, -6.4) normal (0, 0, 1) x (1, 0, 0)
ref_plane "WorkPlane38" through (0, 0, -6.4) normal (0, 0, 1) x (1, 0, 0)
ref_plane "WorkPlane39" through (0, 0, -6.4) normal (0, 0, 1) x (1, 0, 0)
ref_plane "WorkPlane40" through (0, 0, -6.4) normal (0, 0, 1) x (1, 0, 0)
ref_plane "WorkPlane41" through (0, 0, -6.4) normal (0, 0, 1) x (1, 0, 0)
ref_plane "WorkPlane42" through (0, 0, -6.4) normal (0, 0, 1) x (1, 0, 0)
ref_plane "WorkPlane43" through (0, 0, -6.4) normal (0, 0, 1) x (1, 0, 0)
ref_plane "WorkPlane44" through (0, 0, -6.4) normal (0, 0, 1) x (1, 0, 0)
ref_plane "WorkPlane45" through (0, 0, -6.4) normal (0, 0, 1) x (1, 0, 0)
ref_plane "WorkPlane46" through (0, 0, 2) normal (0, 0, 1) x (1, 0, 0)
sketch "CrossOpen" plane through (0, 0, 0) normal (0, 0, 1) x (1, 0, 0)
  line L0 (59, 25.8) -> (96, 25.8)
  line L1 (96, 25.8) -> (96, 38.2)
  line L2 (96, 38.2) -> (59, 38.2)
  line L3 (59, 38.2) -> (59, 25.8)
  line L4 (71.3, 13.5) -> (83.7, 13.5)
  line L5 (83.7, 13.5) -> (83.7, 50.5)
  line L6 (83.7, 50.5) -> (71.3, 50.5)
  line L7 (71.3, 50.5) -> (71.3, 13.5)
ref_plane "WorkPlane47" through (0, 0, -6.4) normal (0, 0, 1) x (1, 0, 0)
ref_plane "WorkPlane48" through (0, 0, -6.4) normal (0, 0, 1) x (1, 0, 0)
ref_plane "WorkPlane49" through (0, 0, -6.4) normal (0, 0, 1) x (1, 0, 0)
ref_plane "WorkPlane50" through (0, 0, 2) normal (0, 0, 1) x (1, 0, 0)
ref_plane "WorkPlane51" through (0, 0, 2) normal (0, 0, 1) x (1, 0, 0)
sketch "dt3_U" plane through (0, 0, 0) normal (0, 0, 1) x (1, 0, 0)
  line L0 (77.5, 44.75) -> (75.25, 40.25)
  line L1 (75.25, 40.25) -> (79.75, 40.25)
  line L2 (79.75, 40.25) -> (77.5, 44.75)
sketch "dt3_D" plane through (0, 0, 0) normal (0, 0, 1) x (1, 0, 0)
  line L0 (77.5, 19.25) -> (79.75, 23.75)
  line L1 (79.75, 23.75) -> (75.25, 23.75)
  line L2 (75.25, 23.75) -> (77.5, 19.25)
sketch "dt3_L" plane through (0, 0, 0) normal (0, 0, 1) x (1, 0, 0)
  line L0 (64.75, 32) -> (69.25, 29.75)
  line L1 (69.25, 29.75) -> (69.25, 34.25)
  line L2 (69.25, 34.25) -> (64.75, 32)
sketch "dt3_R" plane through (0, 0, 0) normal (0, 0, 1) x (1, 0, 0)
  line L0 (90.25, 32) -> (85.75, 34.25)
  line L1 (85.75, 34.25) -> (85.75, 29.75)
  line L2 (85.75, 29.75) -> (90.25, 32)
move_body "Move2" bodies 5 to x (1, 0, 0) y (0, 1, 0) z (0, 0, 1) at (0, 0, -3)
move_body "Move3" bodies 5 to x (1, 0, 0) y (0, 1, 0) z (0, 0, 1) at (0, 0, -4)
sketch "cutboss_222_75" plane through (0, 0, 0) normal (0, 0, 1) x (1, 0, 0)
  circle A0 centre (222, 75) radius 4
extrude "Extrude487" cut sketch "cutboss_222_75" along normal blind 6 from surface at -7 bodies 4
sketch "cutboss_222_9" plane through (0, 0, 0) normal (0, 0, 1) x (1, 0, 0)
  circle A0 centre (222, 9) radius 4
extrude "Extrude488" cut sketch "cutboss_222_9" along normal blind 6 from surface at -7 bodies 4
sketch "cutboss_133_144" plane through (0, 0, 0) normal (0, 0, 1) x (1, 0, 0)
  circle A0 centre (133, 144) radius 4
extrude "Extrude489" cut sketch "cutboss_133_144" along normal blind 6 from surface at -7 bodies 4
sketch "cutboss_133_75" plane through (0, 0, 0) normal (0, 0, 1) x (1, 0, 0)
  circle A0 centre (133, 75) radius 4
extrude "Extrude490" cut sketch "cutboss_133_75" along normal blind 6 from surface at -7 bodies 4
sketch "cutboss_133_9" plane through (0, 0, 0) normal (0, 0, 1) x (1, 0, 0)
  circle A0 centre (133, 9) radius 4
extrude "Extrude491" cut sketch "cutboss_133_9" along normal blind 6 from surface at -7 bodies 4
sketch "cutboss_222_129" plane through (0, 0, 0) normal (0, 0, 1) x (1, 0, 0)
  circle A0 centre (222, 129) radius 4
extrude "Extrude492" cut sketch "cutboss_222_129" along normal blind 6 from surface at -7 bodies 4
sketch "m2b_222_75" plane through (0, 0, 0) normal (0, 0, 1) x (1, 0, 0)
  circle A0 centre (222, 75) radius 0.8
extrude "Extrude505" cut sketch "m2b_222_75" against normal blind 2.2 from surface at -7 bodies 4
sketch "m2b_222_9" plane through (0, 0, 0) normal (0, 0, 1) x (1, 0, 0)
  circle A0 centre (222, 9) radius 0.8
extrude "Extrude506" cut sketch "m2b_222_9" against normal blind 2.2 from surface at -7 bodies 4
sketch "m2b_133_144" plane through (0, 0, 0) normal (0, 0, 1) x (1, 0, 0)
  circle A0 centre (133, 144) radius 0.8
extrude "Extrude507" cut sketch "m2b_133_144" against normal blind 2.2 from surface at -7 bodies 4
sketch "m2b_133_75" plane through (0, 0, 0) normal (0, 0, 1) x (1, 0, 0)
  circle A0 centre (133, 75) radius 0.8
extrude "Extrude508" cut sketch "m2b_133_75" against normal blind 2.2 from surface at -7 bodies 4
sketch "m2b_133_9" plane through (0, 0, 0) normal (0, 0, 1) x (1, 0, 0)
  circle A0 centre (133, 9) radius 0.8
extrude "Extrude509" cut sketch "m2b_133_9" against normal blind 2.2 from surface at -7 bodies 4
sketch "m2b_222_129" plane through (0, 0, 0) normal (0, 0, 1) x (1, 0, 0)
  circle A0 centre (222, 129) radius 0.8
extrude "Extrude510" cut sketch "m2b_222_129" against normal blind 2.2 from surface at -7 bodies 4
sketch "dmy_screen" plane through (0, 0, 0) normal (0, 0, 1) x (1, 0, 0)
  line L0 (140.3, 96.3) -> (215.7, 96.3)
  line L1 (215.7, 96.3) -> (215.7, 125.7)
  line L2 (215.7, 125.7) -> (140.3, 125.7)
  line L3 (140.3, 125.7) -> (140.3, 96.3)
extrude "Extrude518" add sketch "dmy_screen" against normal blind 1.8 from surface at -7 separate body makes body 10
sketch "dmy_btn_0" plane through (0, 0, 0) normal (0, 0, 1) x (1, 0, 0)
  line L0 (157.3, 79.3) -> (168.7, 79.3)
  line L1 (168.7, 79.3) -> (168.7, 90.7)
  line L2 (168.7, 90.7) -> (157.3, 90.7)
  line L3 (157.3, 90.7) -> (157.3, 79.3)
extrude "Extrude519" add sketch "dmy_btn_0" against normal blind 1.8 from surface at -7 separate body makes body 11
sketch "dmy_btn_1" plane through (0, 0, 0) normal (0, 0, 1) x (1, 0, 0)
  line L0 (172.3, 79.3) -> (183.7, 79.3)
  line L1 (183.7, 79.3) -> (183.7, 90.7)
  line L2 (183.7, 90.7) -> (172.3, 90.7)
  line L3 (172.3, 90.7) -> (172.3, 79.3)
extrude "Extrude520" add sketch "dmy_btn_1" against normal blind 1.8 from surface at -7 bodies 11 makes body 12
sketch "dmy_btn_2" plane through (0, 0, 0) normal (0, 0, 1) x (1, 0, 0)
  line L0 (142.3, 79.3) -> (153.7, 79.3)
  line L1 (153.7, 79.3) -> (153.7, 90.7)
  line L2 (153.7, 90.7) -> (142.3, 90.7)
  line L3 (142.3, 90.7) -> (142.3, 79.3)
extrude "Extrude521" add sketch "dmy_btn_2" against normal blind 1.8 from surface at -7 bodies 11 makes body 13
sketch "dmy_btn_3" plane through (0, 0, 0) normal (0, 0, 1) x (1, 0, 0)
  line L0 (187.3, 79.3) -> (198.7, 79.3)
  line L1 (198.7, 79.3) -> (198.7, 90.7)
  line L2 (198.7, 90.7) -> (187.3, 90.7)
  line L3 (187.3, 90.7) -> (187.3, 79.3)
extrude "Extrude522" add sketch "dmy_btn_3" against normal blind 1.8 from surface at -7 bodies 11 makes body 14
sketch "dmy_btn_4" plane through (0, 0, 0) normal (0, 0, 1) x (1, 0, 0)
  line L0 (202.3, 79.3) -> (213.7, 79.3)
  line L1 (213.7, 79.3) -> (213.7, 90.7)
  line L2 (213.7, 90.7) -> (202.3, 90.7)
  line L3 (202.3, 90.7) -> (202.3, 79.3)
extrude "Extrude523" add sketch "dmy_btn_4" against normal blind 1.8 from surface at -7 bodies 11 makes body 15
sketch "dmy_btn_5" plane through (0, 0, 0) normal (0, 0, 1) x (1, 0, 0)
  line L0 (157.3, 64.3) -> (168.7, 64.3)
  line L1 (168.7, 64.3) -> (168.7, 75.7)
  line L2 (168.7, 75.7) -> (157.3, 75.7)
  line L3 (157.3, 75.7) -> (157.3, 64.3)
extrude "Extrude524" add sketch "dmy_btn_5" against normal blind 1.8 from surface at -7 bodies 11 makes body 16
sketch "dmy_btn_6" plane through (0, 0, 0) normal (0, 0, 1) x (1, 0, 0)
  line L0 (187.3, 64.3) -> (198.7, 64.3)
  line L1 (198.7, 64.3) -> (198.7, 75.7)
  line L2 (198.7, 75.7) -> (187.3, 75.7)
  line L3 (187.3, 75.7) -> (187.3, 64.3)
extrude "Extrude525" add sketch "dmy_btn_6" against normal blind 1.8 from surface at -7 bodies 11 makes body 17
sketch "dmy_btn_7" plane through (0, 0, 0) normal (0, 0, 1) x (1, 0, 0)
  line L0 (142.3, 64.3) -> (153.7, 64.3)
  line L1 (153.7, 64.3) -> (153.7, 75.7)
  line L2 (153.7, 75.7) -> (142.3, 75.7)
  line L3 (142.3, 75.7) -> (142.3, 64.3)
extrude "Extrude526" add sketch "dmy_btn_7" against normal blind 1.8 from surface at -7 bodies 11 makes body 18
sketch "dmy_btn_8" plane through (0, 0, 0) normal (0, 0, 1) x (1, 0, 0)
  line L0 (172.3, 64.3) -> (183.7, 64.3)
  line L1 (183.7, 64.3) -> (183.7, 75.7)
  line L2 (183.7, 75.7) -> (172.3, 75.7)
  line L3 (172.3, 75.7) -> (172.3, 64.3)
extrude "Extrude527" add sketch "dmy_btn_8" against normal blind 1.8 from surface at -7 bodies 11 makes body 19
sketch "dmy_btn_9" plane through (0, 0, 0) normal (0, 0, 1) x (1, 0, 0)
  line L0 (202.3, 64.3) -> (213.7, 64.3)
  line L1 (213.7, 64.3) -> (213.7, 75.7)
  line L2 (213.7, 75.7) -> (202.3, 75.7)
  line L3 (202.3, 75.7) -> (202.3, 64.3)
extrude "Extrude528" add sketch "dmy_btn_9" against normal blind 1.8 from surface at -7 bodies 11 makes body 20
sketch "dmy_btn_10" plane through (0, 0, 0) normal (0, 0, 1) x (1, 0, 0)
  line L0 (142.3, 40.3) -> (152.7, 40.3)
  line L1 (152.7, 40.3) -> (152.7, 50.7)
  line L2 (152.7, 50.7) -> (142.3, 50.7)
  line L3 (142.3, 50.7) -> (142.3, 40.3)
extrude "Extrude529" add sketch "dmy_btn_10" against normal blind 1.8 from surface at -7 bodies 11 makes body 21
sketch "dmy_btn_11" plane through (0, 0, 0) normal (0, 0, 1) x (1, 0, 0)
  line L0 (155.3, 40.3) -> (165.7, 40.3)
  line L1 (165.7, 40.3) -> (165.7, 50.7)
  line L2 (165.7, 50.7) -> (155.3, 50.7)
  line L3 (155.3, 50.7) -> (155.3, 40.3)
extrude "Extrude530" add sketch "dmy_btn_11" against normal blind 1.8 from surface at -7 bodies 11 makes body 22
sketch "dmy_btn_12" plane through (0, 0, 0) normal (0, 0, 1) x (1, 0, 0)
  line L0 (203.3, 27.3) -> (213.7, 27.3)
  line L1 (213.7, 27.3) -> (213.7, 38.7)
  line L2 (213.7, 38.7) -> (203.3, 38.7)
  line L3 (203.3, 38.7) -> (203.3, 27.3)
sketch "dmy_btn_13" plane through (0, 0, 0) normal (0, 0, 1) x (1, 0, 0)
  line L0 (139.3, 10.3) -> (164.7, 10.3)
  line L1 (164.7, 10.3) -> (164.7, 20.7)
  line L2 (164.7, 20.7) -> (139.3, 20.7)
  line L3 (139.3, 20.7) -> (139.3, 10.3)
extrude "Extrude532" add sketch "dmy_btn_13" against normal blind 1.8 from surface at -7 bodies 11 makes body 23
sketch "dmy_btn_14" plane through (0, 0, 0) normal (0, 0, 1) x (1, 0, 0)
  line L0 (190.3, 10.3) -> (215.7, 10.3)
  line L1 (215.7, 10.3) -> (215.7, 20.7)
  line L2 (215.7, 20.7) -> (190.3, 20.7)
  line L3 (190.3, 20.7) -> (190.3, 10.3)
extrude "Extrude533" add sketch "dmy_btn_14" against normal blind 1.8 from surface at -7 bodies 11 makes body 24
sketch "dmy_btn_15" plane through (0, 0, 0) normal (0, 0, 1) x (1, 0, 0)
  line L0 (186.3, 46.3) -> (198.7, 46.3)
  line L1 (198.7, 46.3) -> (198.7, 49.7)
  line L2 (198.7, 49.7) -> (186.3, 49.7)
  line L3 (186.3, 49.7) -> (186.3, 46.3)
extrude "Extrude534" add sketch "dmy_btn_15" against normal blind 1.8 from surface at -7 bodies 11 makes body 25
sketch "dmy_btn_16" plane through (0, 0, 0) normal (0, 0, 1) x (1, 0, 0)
  line L0 (202.3, 46.3) -> (214.7, 46.3)
  line L1 (214.7, 46.3) -> (214.7, 49.7)
  line L2 (214.7, 49.7) -> (202.3, 49.7)
  line L3 (202.3, 49.7) -> (202.3, 46.3)
extrude "Extrude535" add sketch "dmy_btn_16" against normal blind 1.8 from surface at -7 bodies 11 makes body 26
ref_plane "WorkPlane52" through (0, 0, -9) normal (0, 0, 1) x (1, 0, 0)
ref_plane "WorkPlane53" through (0, 0, -8.8) normal (0, 0, 1) x (1, 0, 0)
sketch "dflg_Dummy_Screen_R" plane through (0, 0, -8.8) normal (0, 0, 1) x (1, 0, 0)
  line L0 (139.4, 95.4) -> (216.6, 95.4)
  line L1 (216.6, 95.4) -> (216.6, 126.6)
  line L2 (216.6, 126.6) -> (139.4, 126.6)
  line L3 (139.4, 126.6) -> (139.4, 95.4)
extrude "Extrude554" add sketch "dflg_Dummy_Screen_R" against normal blind 1.2 bodies 10
sketch "dflg_DummyKey_Top_157" plane through (0, 0, -8.8) normal (0, 0, 1) x (1, 0, 0)
  line L0 (156.4, 78.4) -> (169.6, 78.4)
  line L1 (169.6, 78.4) -> (169.6, 91.6)
  line L2 (169.6, 91.6) -> (156.4, 91.6)
  line L3 (156.4, 91.6) -> (156.4, 78.4)
extrude "Extrude555" add sketch "dflg_DummyKey_Top_157" against normal blind 1.2 bodies 11